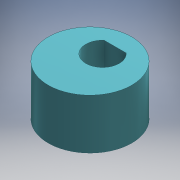
# Autodesk Inventor part: Cam
Saved by Autodesk Inventor 2016 (Build 200138000, 138)
## iProperties
Created: 2015-12-09
Part Number: Cam
Material: Generic
Document SubType Name: Modeling
Designer: lk8187
Density: 1 g/cm^3
Appearance: Smooth - Dark Cadet Blue
Author: lk8187
Autodesk Inventor part; units mm, degrees
ref_plane "YZ Plane" through (0, 0, 0) normal (1, 0, 0) x (0, 1, 0)
ref_plane "XZ Plane" through (0, 0, 0) normal (0, 1, 0) x (-1, 0, 0)
ref_plane "XY Plane" through (0, 0, 0) normal (0, 0, 1) x (1, 0, 0)
sketch "Sketch1" plane through (0, 0, 0) normal (0, 0, 1) x (1, 0, 0)
  arc A0 (-1.3229, 1.5) -> (1.3229, 1.5) centre (0, 0) ccw
  line L0 (-1.3229, 1.5) -> (1.3229, 1.5)
  circle A1 centre (0, -1.5) radius 5
  dimension "d0" = 2
  dimension "d1" = 1.5
  dimension "d2" = 10
  dimension "d3" = 1.5
  constraints: 2 centre point, 2 end point, 2 point on circle, 1 coincident, 1 horizontal, 1 vertical alignment
  measures "d0" radius of A0
  measures "d1" distance from line of L0 point (0, 0)
  measures "d2" diameter of A1
  measures "d3" distance of A1.centre point (0, 0)
extrude "Extrusion1" add sketch "Sketch1" along normal blind 6
body "Solid1"
